Autodesk Inventor part; units mm, degrees
(part 4 of 4)
sketch "스케치48" plane through (0, 0, 0) normal (0, -1, 0) x (1, 0, 0)
  line L0 (15, -83.501) -> (15, -93.501) projected
  arc A0 (13, -95.501) -> (15, -93.501) centre (13, -93.501) ccw projected
  line L1 (13, -95.501) -> (-13, -95.501) projected
  arc A1 (-15, -93.501) -> (-13, -95.501) centre (-13, -93.501) ccw projected
  line L2 (-15, -93.501) -> (-15, -83.501) projected
  arc A2 (-13, -81.501) -> (-15, -83.501) centre (-13, -83.501) ccw projected
  line L3 (-13, -81.501) -> (13, -81.501) projected
  arc A3 (15, -83.501) -> (13, -81.501) centre (13, -83.501) ccw projected
  circle A4 centre (-4.9749, -12.0104) radius 1.6 projected
  circle A5 centre (12.0104, -4.9749) radius 1.6 projected
  circle A6 centre (4.9749, -12.0104) radius 1.6 projected
  circle A7 centre (-12.0104, -4.9749) radius 1.6 projected
  arc A8 (13, 81.501) -> (15, 83.501) centre (13, 83.501) ccw projected
  line L4 (13, 81.501) -> (-13, 81.501) projected
  arc A9 (-15, 83.501) -> (-13, 81.501) centre (-13, 83.501) ccw projected
  line L5 (-15, 83.501) -> (-15, 93.501) projected
  arc A10 (-13, 95.501) -> (-15, 93.501) centre (-13, 93.501) ccw projected
  line L6 (-13, 95.501) -> (13, 95.501) projected
  arc A11 (15, 93.501) -> (13, 95.501) centre (13, 93.501) ccw projected
  line L7 (15, 93.501) -> (15, 83.501) projected
  circle A12 centre (0, 0) radius 8 projected
  circle A13 centre (99.9787, 108.101) radius 1.85 projected
  circle A14 centre (15.7787, -108.101) radius 1.85 projected
  circle A15 centre (35.7787, 108.101) radius 1.75 projected
  circle A16 centre (119.9787, -108.101) radius 1.75 projected
  circle A17 centre (119.9787, 108.101) radius 1.75 projected
  circle A18 centre (35.7787, -108.101) radius 1.75 projected
  circle A19 centre (15.7787, 108.101) radius 1.85 projected
  circle A20 centre (99.9787, -108.101) radius 1.85 projected
  line L8 (50.8787, 118.101) -> (84.8787, 118.101) projected
  arc A21 (87.8787, 115.101) -> (84.8787, 118.101) centre (84.8787, 115.101) ccw projected
  line L9 (87.8787, 115.101) -> (87.8787, 101.101) projected
  arc A22 (84.8787, 98.101) -> (87.8787, 101.101) centre (84.8787, 101.101) ccw projected
  line L10 (84.8787, 98.101) -> (50.8787, 98.101) projected
  arc A23 (47.8787, 101.101) -> (50.8787, 98.101) centre (50.8787, 101.101) ccw projected
  line L11 (47.8787, 101.101) -> (47.8787, 115.101) projected
  arc A24 (50.8787, 118.101) -> (47.8787, 115.101) centre (50.8787, 115.101) ccw projected
  circle A25 centre (114.8107, 128.501) radius 1.6 projected
  circle A26 centre (34.8107, 128.501) radius 1.6 projected
  circle A27 centre (49.8107, 128.501) radius 1.6 projected
  circle A28 centre (89.8107, 128.501) radius 1.6 projected
  circle A29 centre (4.8107, 128.501) radius 1.6 projected
  circle A30 centre (-15.1893, 128.501) radius 1.6 projected
  circle A31 centre (69.8107, 128.501) radius 1.6 projected
  line L12 (84.8787, -118.101) -> (50.8787, -118.101) projected
  arc A32 (47.8787, -115.101) -> (50.8787, -118.101) centre (50.8787, -115.101) ccw projected
  line L13 (47.8787, -115.101) -> (47.8787, -101.101) projected
  arc A33 (50.8787, -98.101) -> (47.8787, -101.101) centre (50.8787, -101.101) ccw projected
  line L14 (50.8787, -98.101) -> (84.8787, -98.101) projected
  arc A34 (87.8787, -101.101) -> (84.8787, -98.101) centre (84.8787, -101.101) ccw projected
  line L15 (87.8787, -101.101) -> (87.8787, -115.101) projected
  arc A35 (84.8787, -118.101) -> (87.8787, -115.101) centre (84.8787, -115.101) ccw projected
  circle A36 centre (12.0104, 4.9749) radius 1.6 projected
  circle A37 centre (-12.0104, 4.9749) radius 1.6 projected
  circle A38 centre (4.9749, 12.0104) radius 1.6 projected
  circle A39 centre (-4.9749, 12.0104) radius 1.6 projected
  circle A40 centre (-15.1893, 76.501) radius 1.6 projected
  circle A41 centre (69.8107, 76.501) radius 1.6 projected
  circle A42 centre (89.8107, 76.501) radius 1.6 projected
  circle A43 centre (4.8107, 76.501) radius 1.6 projected
  circle A44 centre (49.8107, 76.501) radius 1.6 projected
  circle A45 centre (114.8107, 76.501) radius 1.6 projected
  circle A46 centre (34.8107, 76.501) radius 1.6 projected
  circle A47 centre (34.8107, -76.501) radius 1.6 projected
  circle A48 centre (114.8107, -76.501) radius 1.6 projected
  circle A49 centre (49.8107, -76.501) radius 1.6 projected
  circle A50 centre (4.8107, -76.501) radius 1.6 projected
  circle A51 centre (89.8107, -76.501) radius 1.6 projected
  circle A52 centre (69.8107, -76.501) radius 1.6 projected
  circle A53 centre (-15.1893, -76.501) radius 1.6 projected
  circle A54 centre (69.8107, -128.501) radius 1.6 projected
  circle A55 centre (-15.1893, -128.501) radius 1.6 projected
  circle A56 centre (4.8107, -128.501) radius 1.6 projected
  circle A57 centre (89.8107, -128.501) radius 1.6 projected
  circle A58 centre (49.8107, -128.501) radius 1.6 projected
  circle A59 centre (34.8107, -128.501) radius 1.6 projected
  circle A60 centre (114.8107, -128.501) radius 1.6 projected
  circle A61 centre (17.9, 59.001) radius 1.6 projected
  circle A62 centre (-18.1, 59.001) radius 1.6 projected
  arc A63 (-30.2213, -120.9669) -> (-18.2213, -132.9669) centre (-18.2213, -120.9669) ccw projected
  line L16 (-18.2213, -132.9669) -> (115.7787, -132.9669) projected
  arc A64 (115.7787, -132.9669) -> (127.7787, -120.9669) centre (115.7787, -120.9669) ccw projected
  line L17 (127.7787, -120.9669) -> (127.7787, -81.2883) projected
  arc A65 (127.7787, -81.2883) -> (120.2094, -70.1362) centre (115.7787, -81.2883) ccw projected
  line L18 (120.2094, -70.1362) -> (38.4539, -37.6545) projected
  arc A66 (34.7638, -33.1392) -> (38.4539, -37.6545) centre (40.6692, -32.0784) ccw projected
  arc A67 (34.7638, -33.1392) -> (28.8583, -28.2) centre (28.8583, -34.2) ccw projected
  line L19 (28.8583, -28.2) -> (27.1, -28.2) projected
  line L20 (27.1, -28.2) -> (27.1, 28.2) projected
  line L21 (27.1, 28.2) -> (28.8583, 28.2) projected
  arc A68 (28.8583, 28.2) -> (34.7638, 33.1392) centre (28.8583, 34.2) ccw projected
  arc A69 (38.4539, 37.6545) -> (34.7638, 33.1392) centre (40.6692, 32.0784) ccw projected
  line L22 (38.4539, 37.6545) -> (120.2094, 70.1362) projected
  arc A70 (120.2094, 70.1362) -> (127.7787, 81.2883) centre (115.7787, 81.2883) ccw projected
  line L23 (127.7787, 81.2883) -> (127.7787, 120.9669) projected
  arc A71 (127.7787, 120.9669) -> (115.7787, 132.9669) centre (115.7787, 120.9669) ccw projected
  line L24 (115.7787, 132.9669) -> (-18.2213, 132.9669) projected
  arc A72 (-18.2213, 132.9669) -> (-30.2213, 120.9669) centre (-18.2213, 120.9669) ccw projected
  line L25 (-30.2213, 120.9669) -> (-30.2213, 28.2) projected
  line L26 (-30.2213, 28.2) -> (-27.1, 28.2) projected
  line L27 (-27.1, 28.2) -> (-27.1, -28.2) projected
  line L28 (-27.1, -28.2) -> (-30.2213, -28.2) projected
  line L29 (-30.2213, -28.2) -> (-30.2213, -120.9669) projected
  line L30 (-30.2213, -120.9669) -> (-30.2213, -28.2) projected
  line L31 (-30.2213, -120.9669) -> (-30.2213, -150)
  line L32 (-30.2213, 120.9669) -> (-30.2213, 28.2) projected
  line L33 (-30.2213, 120.9669) -> (-30.2213, 150)
  line L34 (-30.2213, -150) -> (127.7787, -150)
  arc A73 (115.7787, -132.9669) -> (127.7787, -120.9669) centre (115.7787, -120.9669) ccw projected
  line L35 (127.7787, -150) -> (127.7787, -120.9669)
  line L36 (-30.2213, 150) -> (127.7787, 150)
  line L37 (127.7787, 150) -> (127.7787, 120.9669)
  dimension "d338" = 300
  dimension "d340" = 150
  constraints: 12 end point, 2 horizontal, 2 perpendicular, 2 tangent, 2 vertical
  measures "d338" distance of L31.end L33.end
  measures "d340" vertical distance of point (0, 0) L31.end
extrude "돌출48" add sketch "스케치48" against normal blind 5 contours A63 L16 A64 L35 L34 L31 | L33 L36 L37 A71 L24 A72
sketch "스케치49" plane through (0, 0, 0) normal (0, -1, 0) x (1, 0, 0)
  line L0 (15, -83.501) -> (15, -93.501) projected
  arc A0 (13, -95.501) -> (15, -93.501) centre (13, -93.501) ccw projected
  line L1 (13, -95.501) -> (-13, -95.501) projected
  arc A1 (-15, -93.501) -> (-13, -95.501) centre (-13, -93.501) ccw projected
  line L2 (-15, -93.501) -> (-15, -83.501) projected
  arc A2 (-13, -81.501) -> (-15, -83.501) centre (-13, -83.501) ccw projected
  line L3 (-13, -81.501) -> (13, -81.501) projected
  arc A3 (15, -83.501) -> (13, -81.501) centre (13, -83.501) ccw projected
  circle A4 centre (-4.9749, -12.0104) radius 1.6 projected
  circle A5 centre (12.0104, -4.9749) radius 1.6 projected
  circle A6 centre (4.9749, -12.0104) radius 1.6 projected
  circle A7 centre (-12.0104, -4.9749) radius 1.6 projected
  arc A8 (13, 81.501) -> (15, 83.501) centre (13, 83.501) ccw projected
  line L4 (13, 81.501) -> (-13, 81.501) projected
  arc A9 (-15, 83.501) -> (-13, 81.501) centre (-13, 83.501) ccw projected
  line L5 (-15, 83.501) -> (-15, 93.501) projected
  arc A10 (-13, 95.501) -> (-15, 93.501) centre (-13, 93.501) ccw projected
  line L6 (-13, 95.501) -> (13, 95.501) projected
  arc A11 (15, 93.501) -> (13, 95.501) centre (13, 93.501) ccw projected
  line L7 (15, 93.501) -> (15, 83.501) projected
  circle A12 centre (0, 0) radius 8 projected
  circle A13 centre (99.9787, 108.101) radius 1.85 projected
  circle A14 centre (15.7787, -108.101) radius 1.85 projected
  circle A15 centre (35.7787, 108.101) radius 1.75 projected
  circle A16 centre (119.9787, -108.101) radius 1.75 projected
  circle A17 centre (119.9787, 108.101) radius 1.75 projected
  circle A18 centre (35.7787, -108.101) radius 1.75 projected
  circle A19 centre (15.7787, 108.101) radius 1.85 projected
  circle A20 centre (99.9787, -108.101) radius 1.85 projected
  line L8 (50.8787, 118.101) -> (84.8787, 118.101) projected
  arc A21 (87.8787, 115.101) -> (84.8787, 118.101) centre (84.8787, 115.101) ccw projected
  line L9 (87.8787, 115.101) -> (87.8787, 101.101) projected
  arc A22 (84.8787, 98.101) -> (87.8787, 101.101) centre (84.8787, 101.101) ccw projected
  line L10 (84.8787, 98.101) -> (50.8787, 98.101) projected
  arc A23 (47.8787, 101.101) -> (50.8787, 98.101) centre (50.8787, 101.101) ccw projected
  line L11 (47.8787, 101.101) -> (47.8787, 115.101) projected
  arc A24 (50.8787, 118.101) -> (47.8787, 115.101) centre (50.8787, 115.101) ccw projected
  circle A25 centre (114.8107, 128.501) radius 1.6 projected
  circle A26 centre (34.8107, 128.501) radius 1.6 projected
  circle A27 centre (49.8107, 128.501) radius 1.6 projected
  circle A28 centre (89.8107, 128.501) radius 1.6 projected
  circle A29 centre (4.8107, 128.501) radius 1.6 projected
  circle A30 centre (-15.1893, 128.501) radius 1.6 projected
  circle A31 centre (69.8107, 128.501) radius 1.6 projected
  line L12 (84.8787, -118.101) -> (50.8787, -118.101) projected
  arc A32 (47.8787, -115.101) -> (50.8787, -118.101) centre (50.8787, -115.101) ccw projected
  line L13 (47.8787, -115.101) -> (47.8787, -101.101) projected
  arc A33 (50.8787, -98.101) -> (47.8787, -101.101) centre (50.8787, -101.101) ccw projected
  line L14 (50.8787, -98.101) -> (84.8787, -98.101) projected
  arc A34 (87.8787, -101.101) -> (84.8787, -98.101) centre (84.8787, -101.101) ccw projected
  line L15 (87.8787, -101.101) -> (87.8787, -115.101) projected
  arc A35 (84.8787, -118.101) -> (87.8787, -115.101) centre (84.8787, -115.101) ccw projected
  circle A36 centre (12.0104, 4.9749) radius 1.6 projected
  circle A37 centre (-12.0104, 4.9749) radius 1.6 projected
  circle A38 centre (4.9749, 12.0104) radius 1.6 projected
  circle A39 centre (-4.9749, 12.0104) radius 1.6 projected
  circle A40 centre (-15.1893, 76.501) radius 1.6 projected
  circle A41 centre (69.8107, 76.501) radius 1.6 projected
  circle A42 centre (89.8107, 76.501) radius 1.6 projected
  circle A43 centre (4.8107, 76.501) radius 1.6 projected
  circle A44 centre (49.8107, 76.501) radius 1.6 projected
  circle A45 centre (114.8107, 76.501) radius 1.6 projected
  circle A46 centre (34.8107, 76.501) radius 1.6 projected
  circle A47 centre (34.8107, -76.501) radius 1.6 projected
  circle A48 centre (114.8107, -76.501) radius 1.6 projected
  circle A49 centre (49.8107, -76.501) radius 1.6 projected
  circle A50 centre (4.8107, -76.501) radius 1.6 projected
  circle A51 centre (89.8107, -76.501) radius 1.6 projected
  circle A52 centre (69.8107, -76.501) radius 1.6 projected
  circle A53 centre (-15.1893, -76.501) radius 1.6 projected
  circle A54 centre (69.8107, -128.501) radius 1.6 projected
  circle A55 centre (-15.1893, -128.501) radius 1.6 projected
  circle A56 centre (4.8107, -128.501) radius 1.6 projected
  circle A57 centre (89.8107, -128.501) radius 1.6 projected
  circle A58 centre (49.8107, -128.501) radius 1.6 projected
  circle A59 centre (34.8107, -128.501) radius 1.6 projected
  circle A60 centre (114.8107, -128.501) radius 1.6 projected
  circle A61 centre (17.9, 59.001) radius 1.6 projected
  circle A62 centre (-18.1, 59.001) radius 1.6 projected
  line L16 (-30.2213, -28.2) -> (-30.2213, -150) projected
  line L17 (-30.2213, -150) -> (127.7787, -150) projected
  line L18 (127.7787, -150) -> (127.7787, -81.2883) projected
  arc A63 (127.7787, -81.2883) -> (120.2094, -70.1362) centre (115.7787, -81.2883) ccw projected
  line L19 (120.2094, -70.1362) -> (38.4539, -37.6545) projected
  arc A64 (34.7638, -33.1392) -> (38.4539, -37.6545) centre (40.6692, -32.0784) ccw projected
  arc A65 (34.7638, -33.1392) -> (28.8583, -28.2) centre (28.8583, -34.2) ccw projected
  line L20 (28.8583, -28.2) -> (27.1, -28.2) projected
  line L21 (27.1, -28.2) -> (27.1, 28.2) projected
  line L22 (27.1, 28.2) -> (28.8583, 28.2) projected
  arc A66 (28.8583, 28.2) -> (34.7638, 33.1392) centre (28.8583, 34.2) ccw projected
  arc A67 (38.4539, 37.6545) -> (34.7638, 33.1392) centre (40.6692, 32.0784) ccw projected
  line L23 (38.4539, 37.6545) -> (120.2094, 70.1362) projected
  arc A68 (120.2094, 70.1362) -> (127.7787, 81.2883) centre (115.7787, 81.2883) ccw projected
  line L24 (127.7787, 81.2883) -> (127.7787, 150) projected
  line L25 (127.7787, 150) -> (-30.2213, 150) projected
  line L26 (-30.2213, 150) -> (-30.2213, 28.2) projected
  line L27 (-30.2213, 28.2) -> (-27.1, 28.2) projected
  line L28 (-27.1, 28.2) -> (-27.1, -28.2) projected
  line L29 (-27.1, -28.2) -> (-30.2213, -28.2) projected
  circle A69 centre (-15.1893, -128.501) radius 1.6
  circle A70 centre (4.8107, -128.501) radius 1.6 projected
  circle A71 centre (4.8107, -128.501) radius 1.6
  circle A72 centre (34.8107, -128.501) radius 1.6
  circle A73 centre (-15.1893, -128.501) radius 1.6 projected
  line L30 (-15.1893, -128.501) -> (-15.1893, -146.101)
  circle A74 centre (-15.1893, -146.101) radius 1.6
  circle A75 centre (4.8107, -146.101) radius 1.6
  circle A76 centre (34.8107, -146.101) radius 1.6
  circle A77 centre (49.8107, -146.101) radius 1.6
  circle A78 centre (69.8107, -146.101) radius 1.6
  circle A79 centre (89.8107, -146.101) radius 1.6
  circle A80 centre (114.8107, -146.101) radius 1.6
  dimension "d343" = 17.6
  dimension "d344" = 3.2
  constraints: 10 centre point, 8 equal radius, 6 horizontal alignment, 6 vertical alignment, 4 coincident, 2 end point, 1 vertical
  measures "d343" distance of L30.start L30.end
  measures "d344" diameter of A74
extrude "돌출49" add sketch "스케치49" against normal blind 5 contours A54 | A55 | A56 | A57 | A58 | A59 | A60
extrude "돌출50" cut sketch "스케치49" against normal blind 5 contours A74 | A75 | A76 | A77 | A78 | A79 | A80
mirror "미러5" about plane through (0, 0, 0) normal (0, 0, 1) of "돌출50"
mirror "미러6" about plane through (0, 0, 0) normal (0, 0, 1) of "돌출49"
fillet "모깎기11" radius 12 4 edges at (-30.2213, 2.5, 150) (-30.2213, 2.5, -150) (127.7787, 2.5, -150) (127.7787, 2.5, 150)
equation "\"d2\" = 0.5 * d0"
equation "\"d3\" = 0.5 * d1"
